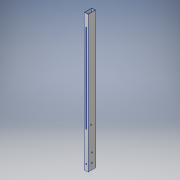
# Autodesk Inventor part: OuterTube
Saved by Autodesk Inventor 2016 SP1 (Build 200210100, 210)
## iProperties
Created: 2016-01-26
Part Number: OuterTube
Material: Aluminum 6061
Document SubType Name: Modeling
Designer: steele
Density: 2.7 g/cm^3
Appearance: Aluminum - Flat
Mass: 1311.66 g
Surface Area: 3189.33 cm^2
Volume: 485.799 cm^3
Author: steele
Autodesk Inventor part; units mm, degrees
ref_plane "YZ Plane" through (0, 0, 0) normal (1, 0, 0) x (0, 1, 0)
ref_plane "XZ Plane" through (0, 0, 0) normal (0, 1, 0) x (-1, 0, 0)
ref_plane "XY Plane" through (0, 0, 0) normal (0, 0, 1) x (1, 0, 0)
sketch "Sketch1" plane through (0, 0, 0) normal (0, 1, 0) x (-1, 0, 0)
  line L0 (15.875, 31.75) -> (-15.875, 31.75)
  line L1 (-15.875, 31.75) -> (-15.875, -31.75)
  line L2 (-15.875, -31.75) -> (15.875, -31.75)
  line L3 (15.875, -31.75) -> (15.875, 31.75)
  line L4 (15.875, 31.75) -> (-15.875, -31.75) construction
  line L5 (-15.875, 31.75) -> (15.875, -31.75) construction
  line L6 (12.7, 28.575) -> (-12.7, 28.575)
  line L7 (-12.7, 28.575) -> (-12.7, -28.575)
  line L8 (-12.7, -28.575) -> (12.7, -28.575)
  line L9 (12.7, -28.575) -> (12.7, 28.575)
  line L10 (12.7, 28.575) -> (-12.7, -28.575) construction
  line L11 (-12.7, 28.575) -> (12.7, -28.575) construction
  point P0 (0, 0)
  dimension "d0" = 63.5
  dimension "d1" = 3.175
  dimension "d26" = 3.175
  dimension "d27" = 31.75
  constraints: 24 end point, 4 midpoint, 2 horizontal, 2 perpendicular, 1 parallel, 1 vertical
  measures "d0" distance of L2.end L0.start
  measures "d1" distance between parallel lines of L6 L0
  measures "d26" distance between parallel lines of L9 L3
  measures "d27" distance of L0.start L0.end
extrude "Extrusion1" add sketch "Sketch1" along normal blind 1143
sketch "Sketch4" plane through (-15.875, 0, 31.75) normal (0, 0, 1) x (1, 0, 0)
  line L0 (15.875, 0) -> (15.875, 1143) construction
  line L1 (15.875, 304.8) -> (15.875, 1041.4) construction
  line L2 (19.05, 304.8) -> (19.05, 1041.4)
  line L3 (12.7, 1041.4) -> (12.7, 304.8)
  arc A0 (12.7, 304.8) -> (19.05, 304.8) centre (15.875, 304.8) ccw
  arc A1 (19.05, 1041.4) -> (12.7, 1041.4) centre (15.875, 1041.4) ccw
  line L4 (0, 1143) -> (31.75, 1143) projected
  line L5 (0, 0) -> (31.75, 0) projected
  point P0 (15.875, 673.1)
  dimension "d6" = 6.35
  dimension "d7" = 101.6
  dimension "d8" = 304.8
  dimension "d28" = 736.6
  constraints: 10 end point, 4 point on circle, 4 tangent, 2 centre point, 2 point on line, 1 midpoint, 1 parallel, 1 vertical
  measures "d6" distance between parallel lines of L2 L3
  measures "d7" distance from line of L2.end L4
  measures "d8" distance from line of L2.start L5
  measures "d28" distance of L1.end L1.start
extrude "Extrusion3" cut sketch "Sketch4" against normal through all
sketch "Sketch5" plane through (15.875, 0, 31.75) normal (1, 0, 0) x (0, 0, -1)
  circle A0 centre (31.75, 127) radius 4.7625
  line L0 (0, 0) -> (63.5, 0) projected
  line L1 (0, 0) -> (0, 1143) projected
  point P0 (31.75, 0)
  dimension "d11" = 9.525
  dimension "d12" = 127
  dimension "d25" = 31.75
  constraints: 1 centre point
  measures "d11" diameter of A0
  measures "d12" distance from line of A0.centre L0
  measures "d25" distance from line of A0.centre L1
extrude "Extrusion4" cut sketch "Sketch5" against normal up to next
sketch "Sketch6" plane through (-15.875, 0, 31.75) normal (0, 0, 1) x (1, 0, 0)
  circle A0 centre (15.875, 50.8) radius 4.7625
  line L0 (0, 0) -> (31.75, 0) projected
  line L1 (0, 0) -> (0, 1143) projected
  point P0 (15.875, 0)
  dimension "d15" = 9.525
  dimension "d16" = 50.8
  dimension "d24" = 15.875
  constraints: 1 centre point
  measures "d15" diameter of A0
  measures "d16" distance from line of A0.centre L0
  measures "d24" distance from line of A0.centre L1
extrude "Extrusion5" cut sketch "Sketch6" against normal through all
sketch "Sketch7" plane through (15.875, 0, 31.75) normal (1, 0, 0) x (0, 0, -1)
  circle A0 centre (31.75, 50.8) radius 4.7625
  line L0 (0, 0) -> (63.5, 0) projected
  line L1 (31.75, 0) -> (31.75, 96.4703) construction
  line L2 (0, 0) -> (0, 1143) construction
  dimension "d19" = 9.525
  dimension "d20" = 50.8
  dimension "d23" = 31.75
  constraints: 2 end point, 1 centre point, 1 vertical
  measures "d19" diameter of A0
  measures "d20" distance from line of A0.centre L0
  measures "d23" distance from line of A0.centre L2
extrude "Extrusion6" cut sketch "Sketch7" against normal through all
sketch "Sketch8" plane through (15.875, 0, 31.75) normal (1, 0, 0) x (0, 0, -1)
  circle A0 centre (25.4, 330.2) radius 4.7625
  line L0 (0, 1143) -> (63.5, 1143) projected
  point P0 (31.75, 0)
  dimension "d29" = 9.525
  dimension "d30" = 812.8
  constraints: 1 centre point
  measures "d29" diameter of A0
  measures "d30" distance from line of A0.centre L0
extrude "Extrusion7" cut sketch "Sketch8" against normal through all
equation "\"d0\" = tubeBreadth"
equation "\"d1\" = tubeThickness"
equation "\"d27\" = tubeWidth"
equation "\"d2\" = tubeLength"
equation "\"d6\" = slotWidth"
equation "\"d7\" = slotDistanceFromTop"
equation "\"d8\" = slotDistanceFromBottom"
equation "\"d25\" = 0.5 * tubeBreadth"
equation "\"d15\" = axelDiam"
equation "\"d16\" = axelHeightAboveBottomOfTube"
equation "\"d24\" = 0.5 * tubeWidth"
equation "\"d19\" = axelDiam"
equation "\"d20\" = axelHeightAboveBottomOfTube"
equation "\"d23\" = 0.5 * tubeBreadth"
equation "\"d29\" = stopHoleDiam"
equation "\"d30\" = stopHoleDistanceFromTop"
equation "\"tubeBreadth\" = 63.5"
equation "\"tubeThickness\" = 3.175"
equation "\"tubeLength\" = 1143"
equation "\"slotDistanceFromBottom\" = 304.8"
equation "\"slotDistanceFromTop\" = 101.6"
equation "\"slotWidth\" = 6.35"
equation "\"axelDiam\" = 9.525"
equation "\"axelHeightAboveBottomOfTube\" = 50.8"
equation "\"tubeWidth\" = 31.75"
equation "\"stopHoleDiam\" = 9.525"
equation "\"stopHoleDistanceFromTop\" = 812.8"
body "Solid1"
